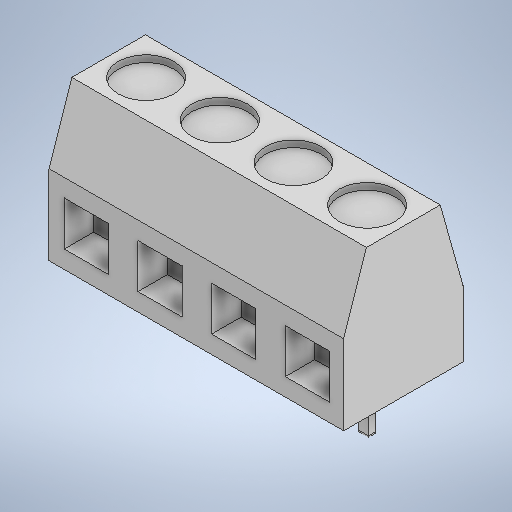
# Autodesk Inventor part: Schraubklemme_1x3
Saved by Autodesk Inventor 2025.1 (Build 291241020, 241B)
## iProperties
Created: 2025-04-15
Part Number: Schraubklemme_1x3
Material: Generisch
Document SubType Name: Modeling
Designer: mexen
Density: 1 g/cm^3
Appearance: Vorgabe
Author: mexen
Autodesk Inventor part; units mm, degrees
ref_plane "YZ Plane" through (0, 0, 0) normal (1, 0, 0) x (0, 1, 0)
ref_plane "XZ Plane" through (0, 0, 0) normal (0, 1, 0) x (-1, 0, 0)
ref_plane "XY Plane" through (0, 0, 0) normal (0, 0, 1) x (1, 0, 0)
sketch "Skizze1" plane through (0, 0, 0) normal (0, 0, 1) x (1, 0, 0)
  line L0 (-10, -4.05) -> (10, -4.05)
  line L1 (10, -4.05) -> (10, 4.05)
  line L2 (10, 4.05) -> (-10, 4.05)
  line L3 (-10, 4.05) -> (-10, -4.05)
  line L4 (-10, -4.05) -> (10, 4.05) construction
  line L5 (10, -4.05) -> (-10, 4.05) construction
  point P0 (0, 0)
  dimension "d0" = 20
  dimension "d1" = 8.1
  constraints: 12 end point, 2 midpoint, 2 parallel, 1 horizontal, 1 perpendicular
  measures "d0" distance of L2.end L1.end
  measures "d1" distance of L1.end L0.end
extrude "Extrusion1" add sketch "Skizze1" along normal blind 10
sketch "Skizze2" plane through (0, 0, 10) normal (0, 0, 1) x (1, 0, 0)
  circle A0 centre (-7.46, 0) radius 1.9
  circle A1 centre (-2.46, 0) radius 1.9
  line L0 (-10, 4.05) -> (-10, -4.05) projected
  circle A2 centre (2.54, 0) radius 1.9
  circle A3 centre (7.54, 0) radius 1.9
  point P0 (0, 0)
  point P1 (-10, 0)
  dimension "d6" = 3.8
  dimension "d7" = 3.8
  dimension "d56" = 2.54
  dimension "d57" = 5
  dimension "d58" = 3.8
  dimension "d59" = 3.8
  dimension "d60" = 5
  dimension "d61" = 5
  constraints: 4 centre point, 1 midpoint
  measures "d6" diameter of A0
  measures "d7" diameter of A1
  measures "d56" distance of point (-10, 0) A0.centre
  measures "d57" distance of A0.centre A1.centre
  measures "d58" diameter of A2
  measures "d59" diameter of A3
  measures "d60" distance of A2.centre A1.centre
  measures "d61" distance of A3.centre A2.centre
extrude "Extrusion2" cut sketch "Skizze2" against normal blind 0.45
chamfer "Fasen1" distance 1.55 distance2 4.59 1 edges at (0, -4.05, 10) measured on face at (-0.7437, -3.3287, 10)
chamfer "Fasen2" distance 1.55 distance2 5.5 1 edges at (0, 4.05, 10) measured on face at (0.7703, 3.3287, 10)
sketch "Skizze3" plane through (0, 0, 0) normal (0, 0, -1) x (-1, 0, 0)
  line L0 (2.81, 0.25) -> (2.11, 0.25)
  line L1 (2.11, 0.25) -> (2.11, -0.25)
  line L2 (2.11, -0.25) -> (2.81, -0.25)
  line L3 (2.81, -0.25) -> (2.81, 0.25)
  line L4 (2.81, 0.25) -> (2.11, -0.25) construction
  line L5 (2.11, 0.25) -> (2.81, -0.25) construction
  line L6 (7.11, 0.25) -> (7.81, 0.25)
  line L7 (7.81, 0.25) -> (7.81, -0.25)
  line L8 (7.81, -0.25) -> (7.11, -0.25)
  line L9 (7.11, -0.25) -> (7.11, 0.25)
  line L10 (7.11, 0.25) -> (7.81, -0.25) construction
  line L11 (7.81, 0.25) -> (7.11, -0.25) construction
  line L12 (10, 4.05) -> (10, -4.05) projected
  line L13 (-2.19, -0.25) -> (-2.89, -0.25)
  line L14 (-2.89, -0.25) -> (-2.89, 0.25)
  line L15 (-2.89, 0.25) -> (-2.19, 0.25)
  line L16 (-2.19, 0.25) -> (-2.19, -0.25)
  line L17 (-2.19, -0.25) -> (-2.89, 0.25) construction
  line L18 (-2.89, -0.25) -> (-2.19, 0.25) construction
  line L19 (-7.19, -0.25) -> (-7.89, -0.25)
  line L20 (-7.89, -0.25) -> (-7.89, 0.25)
  line L21 (-7.89, 0.25) -> (-7.19, 0.25)
  line L22 (-7.19, 0.25) -> (-7.19, -0.25)
  line L23 (-7.19, -0.25) -> (-7.89, 0.25) construction
  line L24 (-7.89, -0.25) -> (-7.19, 0.25) construction
  point P0 (2.46, 0)
  point P1 (7.46, 0)
  point P2 (-2.54, 0)
  point P3 (-7.54, 0)
  dimension "d18" = 0.7
  dimension "d19" = 0.5
  dimension "d20" = 0.7
  dimension "d21" = 0.5
  dimension "d43" = 2.54
  dimension "d45" = 5
  dimension "d48" = 0.7
  dimension "d49" = 0.5
  dimension "d50" = 5
  dimension "d51" = 0.7
  dimension "d52" = 0.5
  dimension "d53" = 5
  constraints: 48 end point, 8 midpoint, 8 parallel, 4 horizontal, 4 perpendicular
  measures "d18" distance of L2.end L1.end
  measures "d19" distance of L1.end L0.end
  measures "d20" distance of L7.end L8.end
  measures "d21" distance of L6.end L7.end
  measures "d43" distance from line of L12 point (7.46, 0)
  measures "d45" distance of point (7.46, 0) point (2.46, 0)
  measures "d48" distance of L14.end L15.end
  measures "d49" distance of L13.end L14.end
  measures "d50" distance of point (-2.54, 0) point (2.46, 0)
  measures "d51" distance of L20.end L21.end
  measures "d52" distance of L19.end L20.end
  measures "d53" distance of point (-2.54, 0) point (-7.54, 0)
extrude "Extrusion3" add sketch "Skizze3" along normal blind 3.5
fillet "Rundung1" radius 0.25 16 edges at (-7.81, 0, -3.5) (-7.11, 0, -3.5) (-7.46, -0.25, -3.5) (-7.46, 0.25, -3.5) (-2.46, -0.25, -3.5) (-2.81, 0, -3.5) (-2.46, 0.25, -3.5) (-2.11, 0, -3.5) (2.54, -0.25, -3.5) (2.19, 0, -3.5) (2.54, 0.25, -3.5) (2.89, 0, -3.5) (7.54, -0.25, -3.5) (7.89, 0, -3.5) (7.54, 0.25, -3.5) (7.19, 0, -3.5)
sketch "Skizze5" plane through (-10, -4.05, 0) normal (0, -1, 0) x (1, 0, 0)
  line L0 (4.04, 1.205) -> (1.04, 1.205)
  line L1 (1.04, 1.205) -> (1.04, 4.205)
  line L2 (1.04, 4.205) -> (4.04, 4.205)
  line L3 (4.04, 4.205) -> (4.04, 1.205)
  line L4 (4.04, 1.205) -> (1.04, 4.205) construction
  line L5 (1.04, 1.205) -> (4.04, 4.205) construction
  line L6 (6.04, 1.205) -> (9.04, 1.205)
  line L7 (9.04, 1.205) -> (9.04, 4.205)
  line L8 (9.04, 4.205) -> (6.04, 4.205)
  line L9 (6.04, 4.205) -> (6.04, 1.205)
  line L10 (6.04, 1.205) -> (9.04, 4.205) construction
  line L11 (9.04, 1.205) -> (6.04, 4.205) construction
  line L12 (11.04, 1.205) -> (14.04, 1.205)
  line L13 (14.04, 1.205) -> (14.04, 4.205)
  line L14 (14.04, 4.205) -> (11.04, 4.205)
  line L15 (11.04, 4.205) -> (11.04, 1.205)
  line L16 (11.04, 1.205) -> (14.04, 4.205) construction
  line L17 (14.04, 1.205) -> (11.04, 4.205) construction
  line L18 (0, 0) -> (0, 5.41) projected
  line L19 (16.04, 1.205) -> (19.04, 1.205)
  line L20 (19.04, 1.205) -> (19.04, 4.205)
  line L21 (19.04, 4.205) -> (16.04, 4.205)
  line L22 (16.04, 4.205) -> (16.04, 1.205)
  line L23 (16.04, 1.205) -> (19.04, 4.205) construction
  line L24 (19.04, 1.205) -> (16.04, 4.205) construction
  point P0 (10, 0)
  point P1 (2.54, 2.705)
  point P2 (7.54, 2.705)
  point P3 (12.54, 2.705)
  point P4 (17.54, 2.705)
  dimension "d27" = 3
  dimension "d28" = 3
  dimension "d29" = 3
  dimension "d30" = 3
  dimension "d31" = 3
  dimension "d32" = 3
  dimension "d33" = 2.54
  dimension "d34" = 5
  dimension "d35" = 5
  dimension "d40" = 3
  dimension "d41" = 3
  dimension "d42" = 5
  constraints: 48 end point, 8 midpoint, 8 parallel, 4 horizontal, 4 perpendicular
  measures "d27" distance of L1.end L2.end
  measures "d28" distance of L0.end L1.end
  measures "d29" distance of L8.end L7.end
  measures "d30" distance of L7.end L6.end
  measures "d31" distance of L14.end L13.end
  measures "d32" distance of L13.end L12.end
  measures "d33" distance from line of L18 point (2.54, 2.705)
  measures "d34" distance of point (7.54, 2.705) point (2.54, 2.705)
  measures "d35" distance of point (12.54, 2.705) point (7.54, 2.705)
  measures "d40" distance of L21.end L20.end
  measures "d41" distance of L20.end L19.end
  measures "d42" distance of point (17.54, 2.705) point (12.54, 2.705)
extrude "Extrusion5" cut sketch "Skizze5" against normal blind 2
